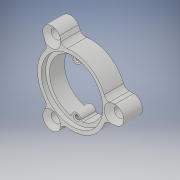
# Autodesk Inventor part: as5047_holder_adder_5mm
Saved by Autodesk Inventor 2019.4 (Build 234330000, 330)
## iProperties
Created: 2019-09-05
Part Number: as5047_holder_adder_5mm
Material: Generic
Document SubType Name: Modeling
Designer: cdi
Density: 1 g/cm^3
Appearance: Default
Author: cdi
Autodesk Inventor part; units mm, degrees
ref_plane "YZ Plane" through (0, 0, 0) normal (1, 0, 0) x (0, 1, 0)
ref_plane "XZ Plane" through (0, 0, 0) normal (0, 1, 0) x (-1, 0, 0)
ref_plane "XY Plane" through (0, 0, 0) normal (0, 0, 1) x (1, 0, 0)
sketch "Sketch1" plane through (0, 0, 0) normal (0, 0, 1) x (1, 0, 0)
  circle A0 centre (0, 0) radius 9
  circle A1 centre (0, 0) radius 11.5
  dimension "d1" = 18
  dimension "d4" = 23
  constraints: 2 centre point, 2 coincident
  measures "d1" diameter of A0
  measures "d4" diameter of A1
extrude "Extrusion1" add sketch "Sketch1" along normal blind 5
sketch "Sketch2" plane through (0, 0, 5) normal (0, 0, 1) x (1, 0, 0)
  circle A0 centre (0, 0) radius 10.25
  circle A1 centre (0, 0) radius 11.5 projected
  dimension "d5" = 20.5
  constraints: 1 centre point, 1 coincident
  measures "d5" diameter of A0
extrude "Extrusion2" add sketch "Sketch2" along normal blind 1.5
sketch "Sketch4" plane through (0, 0, 0) normal (0, 0, -1) x (-1, 0, 0)
  arc A0 (-14, 3) -> (-14, -3) centre (-14, 0) ccw
  arc A1 (-11.5, 0) -> (-11.5, 0) centre (0, 0) ccw projected
  line L0 (-14, 3) -> (-11.1018, 3)
  line L1 (-14, -3) -> (-11.1018, -3)
  arc A2 (-11.1018, 3) -> (-11.1018, -3) centre (0, 0) ccw
  dimension "d13" = 14
  dimension "d14" = 6
  constraints: 6 point on circle, 4 end point, 2 centre point, 2 horizontal, 2 tangent
  measures "d13" distance of point (0, 0) A0.centre
  measures "d14" diameter of A0
extrude "Extrusion4" add sketch "Sketch4" against normal up to surface (6.5 mm away) contours L0 A1 L1 A0
pattern_circular "Circular Pattern1" count 3 over 360 about axis through (0, 0, 0) along (0, 0, 1) of "Extrusion4"
sketch "Sketch5" plane through (0, 0, 6.5) normal (0, 0, 1) x (1, 0, 0)
  arc A0 (14, -3) -> (14, 3) centre (14, 0) ccw projected
  circle A1 centre (14, 0) radius 1.5
  point P0 (0, 0)
  dimension "d20" = 3
  constraints: 1 centre point, 1 coincident
  measures "d20" diameter of A1
hole "Hole1" at (14, 0, 6.5) direction (0, 0, -1) diameter 3.2 depth 15 countersink diameter 6.5 countersink angle 90
pattern_circular "Circular Pattern2" count 3 over 360 about axis through (0, 0, 0) along (0, 0, 1) of "Hole1"
fillet "Fillet1" radius 2 6 edges at (11.1018, -3, 3.25) (11.1018, 3, 3.25) (-8.149, 8.1144, 3.25) (-2.9528, 11.1144, 3.25) (-2.9528, -11.1144, 3.25) (-8.149, -8.1144, 3.25)
sketch "Sketch6" plane through (0, 0, 0) normal (0, 0, -1) x (-1, 0, 0)
  circle A0 centre (0, 0) radius 8.5
  circle A1 centre (0, -8.5) radius 1.5
  circle A2 centre (0, 8.5) radius 1.5
  dimension "d32" = 17
  dimension "d33" = 3
  dimension "d34" = 3
  constraints: 3 centre point, 2 point on circle, 1 coincident
  measures "d32" diameter of A0
  measures "d33" diameter of A1
  measures "d34" diameter of A2
extrude "Extrusion5" add sketch "Sketch6" against normal up to surface (5 mm away) contours A2 A0 | A0 A2 | A1 A0 | A0 A1
sketch "Sketch7" plane through (0, 0, 5) normal (0, 0, 1) x (1, 0, 0)
  arc A0 (-1.4505, 8.8824) -> (1.4505, 8.8824) centre (0, 8.5) ccw projected
  arc A1 (1.4505, -8.8824) -> (-1.4505, -8.8824) centre (0, -8.5) ccw projected
  point P0 (0, 0)
hole "Hole2" at (0, 8.5, 5) at (0, -8.5, 5) direction (0, 0, -1) diameter 1.421 depth 7 thread size "M1.8x0.35" class "6H" standard "ISO Metric profile"
fillet "Fillet2" radius 0.5 4 edges at (1.4505, 8.8824, 2.5) (-1.4505, 8.8824, 2.5) (1.4505, -8.8824, 2.5) (-1.4505, -8.8824, 2.5)
chamfer "Chamfer1" distance 0.3 angle 45 2 edges at (0, -7.7895, 5) (0, 9.2105, 5)
body "Solid1"
